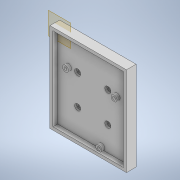
# Autodesk Inventor part: nucleo_din_connector
Saved by Autodesk Inventor 2021 (Build 250183000, 183)
## iProperties
Created: 2020-10-29
Part Number: nucleo_din_connector
Material: Generic
Document SubType Name: Modeling
Designer: Mateusz
Density: 1 g/cm^3
Appearance: Default
Author: Mateusz
Autodesk Inventor part; units mm, degrees
ref_plane "YZ Plane" through (0, 0, 0) normal (1, 0, 0) x (0, 1, 0)
ref_plane "XZ Plane" through (0, 0, 0) normal (0, 1, 0) x (-1, 0, 0)
ref_plane "XY Plane" through (0, 0, 0) normal (0, 0, 1) x (1, 0, 0)
ref_plane "Work Plane1" through (-41.89, 79.898, 0.7952) normal (0, 0, 1) x (1, 0, 0)
sketch "Sketch1" plane through (-41.89, 79.898, 0.7952) normal (0, 0, 1) x (1, 0, 0)
  circle A0 centre (41.89, -79.898) radius 1.45
  circle A1 centre (8.87, -27.828) radius 1.45
  circle A2 centre (57.13, -29.098) radius 1.45
  arc A3 (66, -80.398) -> (68, -78.398) centre (66, -78.398) ccw projected
  line L0 (66, 0.102) -> (0, 0.102) projected
  line L1 (-2, -1.898) -> (-2, -24.398) projected
  line L2 (-2, 0.102) -> (68, 0.102)
  line L3 (68, 0.102) -> (68, -82.398)
  line L4 (68, -82.398) -> (-2, -82.398)
  line L5 (-2, -82.398) -> (-2, 0.102)
  line L6 (-2, 3.102) -> (-5, 3.102)
  line L7 (68, -85.398) -> (71, -85.398)
  line L8 (-5, 3.102) -> (71, 3.102)
  line L9 (71, 3.102) -> (71, -85.398)
  line L10 (71, -85.398) -> (-5, -85.398)
  line L11 (-5, -85.398) -> (-5, 3.102)
  point P0 (44.5, -82.398)
  point P1 (-2, 3.102)
  point P2 (-2, -24.398)
  point P3 (-2, -1.898)
  point P4 (66, 0.102)
  dimension "d0" = 2.9
  dimension "d1" = 2.9
  dimension "d2" = 2.9
  constraints: 20 end point, 4 parallel, 3 centre point, 2 horizontal, 2 perpendicular
  measures "d0" diameter of A0
  measures "d1" diameter of A1
  measures "d2" diameter of A2
extrude "Extrusion1" add sketch "Sketch1" against normal blind 5 contours L2 L3 L4 L5 L1 L0 | L8 L9 L7 L10 L11 L6
sketch "Sketch2" plane through (-41.89, 79.898, 0.7952) normal (0, 0, 1) x (1, 0, 0)
  circle A0 centre (8.87, -27.828) radius 1.45 projected
  circle A1 centre (8.87, -27.828) radius 3
  circle A2 centre (57.13, -29.098) radius 1.45 projected
  circle A3 centre (57.13, -29.098) radius 3
  circle A4 centre (41.89, -79.898) radius 3
  circle A5 centre (41.89, -79.898) radius 1.45
  dimension "d9" = 6
  dimension "d10" = 6
  dimension "d11" = 6
  constraints: 4 centre point, 4 coincident
  measures "d9" diameter of A1
  measures "d10" diameter of A3
  measures "d11" diameter of A4
extrude "Extrusion2" add sketch "Sketch2" along normal blind 3
sketch "Sketch3" plane through (-41.89, 79.898, 0.7952) normal (0, 0, 1) x (1, 0, 0)
  line L0 (71, -85.398) -> (-5, -85.398) projected
  circle A0 centre (18, -27.898) radius 1.45
  circle A1 centre (48, -27.898) radius 1.45
  circle A2 centre (18, -57.898) radius 1.45
  circle A3 centre (48, -57.898) radius 1.45
  point P0 (41.89, -79.898)
  dimension "d19" = 2.9
  dimension "d20" = 2.9
  dimension "d21" = 2.9
  dimension "d22" = 2.9
  constraints: 4 centre point
  measures "d19" diameter of A0
  measures "d20" diameter of A1
  measures "d21" diameter of A2
  measures "d22" diameter of A3
extrude "Extrusion3" cut sketch "Sketch3" against normal up to surface (5 mm away)
sketch "Sketch4" plane through (-41.89, 79.898, 0.7952) normal (0, 0, 1) x (1, 0, 0)
  circle A0 centre (18, -57.898) radius 1.45 projected
  circle A1 centre (18, -57.898) radius 3
  circle A2 centre (18, -57.898) radius 1.45
  circle A3 centre (48, -57.898) radius 1.45 projected
  circle A4 centre (48, -57.898) radius 1.45
  circle A5 centre (48, -57.898) radius 3
  circle A6 centre (48, -27.898) radius 1.45 projected
  circle A7 centre (48, -27.898) radius 1.45
  circle A8 centre (48, -27.898) radius 3
  circle A9 centre (18, -27.898) radius 1.45 projected
  circle A10 centre (18, -27.898) radius 1.45
  circle A11 centre (18, -27.898) radius 3
  point P0 (41.89, -79.898)
  dimension "d25" = 6
  dimension "d26" = 6
  dimension "d27" = 6
  dimension "d28" = 6
  constraints: 8 centre point, 8 coincident
  measures "d25" diameter of A1
  measures "d26" diameter of A5
  measures "d27" diameter of A8
  measures "d28" diameter of A11
extrude "Extrusion4" cut sketch "Sketch4" against normal blind 2
extrude "Extrusion5" add sketch "Sketch1" along normal blind 4.58 contours L8 L9 L7 L10 L11 L6
body "Solid2044"
